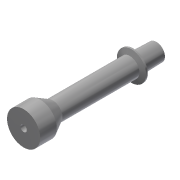
# Autodesk Inventor part: PP-05
Saved by Autodesk Inventor 2022 (Build 260148000, 148)
## iProperties
Created: 2008-09-23
Part Number: PP-05
Document SubType Name: Modeling
Designer: Mark Flayler
Mass: 0.154886 g
Surface Area: 0.785274 cm^2
Volume: 0.0197056 cm^3
Density: 7.86 g/cm^3
Material: Steel, Mild
Description: DISPENSER
Appearance: Steel
Author: Mark Flayler
Autodesk Inventor part; units mm, degrees
ref_plane "YZ Plane" through (0, 0, 0) normal (1, 0, 0) x (0, 1, 0)
ref_plane "XZ Plane" through (0, 0, 0) normal (0, 1, 0) x (-1, 0, 0)
ref_plane "XY Plane" through (0, 0, 0) normal (0, 0, 1) x (1, 0, 0)
sketch "Sketch1" plane through (0, 0, 0) normal (0, 0, 1) x (1, 0, 0)
  line L0 (0, 0) -> (0, 10)
  line L1 (0.24, 0) -> (1.25, 0)
  line L2 (1.25, 0) -> (1.25, 1.25)
  line L3 (1.25, 1.25) -> (0.725, 2.2)
  line L4 (0.725, 2.2) -> (0.725, 8)
  line L5 (0.725, 8) -> (1.1, 8.125)
  line L6 (1.1, 8.125) -> (1.1, 8.25)
  line L7 (1.1, 8.25) -> (0.7, 8.25)
  line L8 (0.7, 8.25) -> (0.65, 10)
  line L9 (0.65, 10) -> (0.3, 10)
  line L10 (0.3, 10) -> (0.24, 0)
  dimension "d1" = 0.25
  dimension "d2" = 0.125
  dimension "d5" = 0.48
  dimension "d6" = 0.6
  dimension "d7" = 2.5
  dimension "d8" = 10
  dimension "d9" = 8
  dimension "d10" = 2.2
  dimension "d11" = 1.25
  dimension "d13" = 2.2
  dimension "d14" = 1.45
  dimension "d15" = 1.3
  dimension "d16" = 1.4
  constraints: 22 end point, 4 parallel, 2 horizontal alignment, 2 perpendicular, 1 vertical
  measures "d1" distance from line of L7 L4.end
  measures "d2" distance of L5.end L6.end
  measures "d5" diameter of L1.start L0
  measures "d6" diameter of L9.end L0
  measures "d7" diameter of L2 L0
  measures "d8" distance from line of L0.start L9
  measures "d9" vertical distance of L0.start L4.end
  measures "d10" vertical distance of L0.start L3.end
  measures "d11" distance of L1.end L2.end
  measures "d13" diameter of L6 L0
  measures "d14" diameter of L4 L0
  measures "d15" diameter of L8.end L0
  measures "d16" diameter of L7.end L0
revolve "Revolution1" add sketch "Sketch1" angle 360 about axis through (0, 0, 0) along (0, 1, 0)
body "Solid1"
